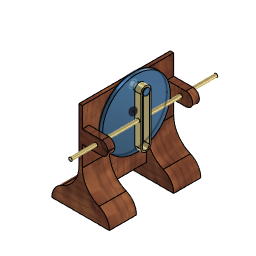
scoci (Autodesk Fusion 360 design; units mm, degrees)
Autodesk Fusion 360 part; units mm, degrees
sketch "Sketch1" plane through (0, 0, 0) normal (1, 0, 0) x (0, 1, 0)
  circle A0 centre (0, 0) radius 50
  circle A1 centre (0, 35) radius 5
  circle A2 centre (0, 0) radius 5
  dimension "d1" = 100
  dimension "d2" = 10
  dimension "d3" = 10
  constraint coincident A0.centre A2.centre
  constraint concentric A0 A2
  measures "d1" diameter of A0
  measures "d2" diameter of A1
  measures "d3" diameter of A2
extrude "Extrude1" add sketch "Sketch1" along normal blind 5 makes body 1
extrude "Extrude2" add sketch "Sketch1" along normal blind 20 contours A1 bodies 1
extrude "Extrude3" add sketch "Sketch1" against normal blind 20 separate body contours A2 makes body 2
extrude "Extrude4" add sketch "Sketch1" along normal blind 5 contours A2 bodies 1 2
ref_plane "WorkPlane1" through (10, 0, 0) normal (1, 0, 0) x (0, 1, 0)
sketch "Sketch2" plane through (10, 0, 0) normal (1, 0, 0) x (0, 1, 0)
  line L0 (-7.4988, -35.1366) -> (-7.5, 34.9999)
  line L1 (7.5, 34.9999) -> (7.5, -35)
  line L2 (-5.25, -35) -> (-5.25, 35)
  line L3 (5.25, -35) -> (5.25, 35)
  arc A0 (-7.4988, -34.8637) -> (7.5, -35) centre (0, -35) ccw
  arc A1 (-5.25, -35) -> (5.25, -35) centre (0, -35) ccw
  arc A2 (7.5, 34.9999) -> (-7.5, 34.9999) centre (0, 35) ccw
  arc A3 (5.25, 35) -> (-5.25, 35) centre (0, 35) ccw
  dimension "d13" = 10.5
  dimension "d14" = 10.5
  dimension "d16" = 15
  constraint concentric A0 A1
  constraint coincident L0.start A0
  constraint tangent L1 A0
  constraint tangent L2 A3
  constraint vertical L2
  constraint tangent L3 A3
  constraint parallel L2 L3
  constraint coincident L0 A0.start
  measures "d13" diameter of A3
  measures "d14" diameter of A1
  measures "d16" diameter of A0
extrude "Extrude5" add sketch "Sketch2" along normal blind 9 separate body makes body 3
sketch "Sketch3" plane through (0, -7.4994, -0.0001) normal (0, -1, -0.000018) x (1, 0, 0)
  line L0 (10, 35) -> (10, -35.1364)
  line L1 (10, -35.1364) -> (19, -35.1364)
  line L2 (19, -35.1364) -> (19, 35)
  line L3 (19, 35) -> (10, 35)
  circle A0 centre (14.92, -0.0682) radius 2.5
  dimension "d19" = 5
  measures "d19" diameter of A0
extrude "Extrude6" add sketch "Sketch3" along normal blind 100 contours A0 bodies 3
sketch "Sketch4" plane through (0, 7.5, 0) normal (0, 1, 0) x (-1, 0, 0)
  line L0 (-10, -35) -> (-10, 34.9999)
  line L1 (-10, 34.9999) -> (-19, 34.9999)
  line L2 (-19, 34.9999) -> (-19, -35)
  line L3 (-19, -35) -> (-10, -35)
  circle A0 centre (-15.0502, -0.0001) radius 2.5
  dimension "d22" = 5
  measures "d22" diameter of A0
extrude "Extrude7" add sketch "Sketch4" along normal blind 100 contours A0 bodies 3
ref_plane "WorkPlane2" through (-5, 0, 0) normal (1, 0, 0) x (0, 1, 0)
sketch "Sketch5" plane through (-5, 0, 0) normal (1, 0, 0) x (0, 1, 0)
  line L0 (65, 40) -> (-70, 40)
  line L1 (-70, 40) -> (-70, -80)
  line L2 (-70, -80) -> (65, -80)
  line L3 (65, -80) -> (65, 40)
  circle A0 centre (0, 0) radius 5.25
  dimension "d26" = 10.5
  constraint horizontal L0
  constraint vertical L1
  constraint horizontal L2
  constraint vertical L3
  constraint coincident A0.centre origin
  measures "d26" diameter of A0
extrude "Extrude8" add sketch "Sketch5" against normal blind 5 separate body makes body 4
sketch "Sketch6" plane through (-5, 0, 0) normal (1, 0, 0) x (0, 1, 0)
  circle A0 centre (0, 0) radius 5.25
  line L0 (65, -80) -> (65, 40)
  line L1 (65, 40) -> (-70, 40)
  line L2 (-70, 40) -> (-70, -80)
  line L3 (-70, -80) -> (65, -80)
  line L4 (-70, -80) -> (-30, -80)
  line L5 (-30, -80) -> (-30, -100)
  line L6 (-30, -100) -> (-70, -100)
  line L7 (-70, -100) -> (-70, -80)
  line L8 (65, -80) -> (25, -80)
  line L9 (25, -80) -> (25, -100)
  line L10 (25, -100) -> (65, -100)
  line L11 (65, -100) -> (65, -80)
  dimension "d29" = 40
  dimension "d30" = 20
  dimension "d31" = 40
  dimension "d32" = 20
  constraint horizontal L4
  constraint vertical L5
  constraint horizontal L6
  constraint vertical L7
  constraint coincident L2.end L3.start
  constraint horizontal L8
  constraint vertical L9
  constraint horizontal L10
  constraint vertical L11
  constraint coincident L0.start L3.end
  measures "d29" distance of L2.end L4.end
  measures "d30" distance of L2.end L6.end
  measures "d31" distance of L0.start L8.end
  measures "d32" distance of L0.start L10.end
extrude "Extrude9" add sketch "Sketch6" against normal blind 45 contours L3 L8 L9 L10 L11 | L3 L4 L5 L6 L7 bodies 4
extrude "Extrude10" add 2 faces at (-50, -56.6667, -86.6667) (-50, 38.3333, -86.6667) along direction (1, 0, 0) blind 85 on bodies 4 bodies 4
fillet "Fillet1" radius 40 4 edges at (-5, -50, -80) (-5, 45, -80) (-10, 45, -80) (-10, -50, -80) on bodies 4
fillet "Fillet2" radius 25 4 edges at (-50, 45, -80) (-50, -50, -80) (35, -50, -80) (35, 45, -80) on bodies 4
sketch "Sketch7" plane through (0, -70, 0) normal (0, -1, 0) x (1, 0, 0)
  arc A0 (35, -100) -> (19.6154, -76.9231) centre (10, -100) ccw
  arc A1 (-5, -40) -> (19.6154, -76.9231) centre (35, -40) ccw
  line L0 (-5, -40) -> (-5, 40)
  line L1 (-5, 40) -> (-10, 40)
  line L2 (-10, 40) -> (-10, -40)
  arc A2 (-34.6154, -76.9231) -> (-10, -40) centre (-50, -40) ccw
  arc A3 (-34.6154, -76.9231) -> (-50, -100) centre (-25, -100) ccw
  line L3 (-50, -100) -> (35, -100)
  line L4 (-5, 9.928) -> (24.1986, 9.928)
  line L5 (33, 0.036) -> (33, -0.036)
  line L6 (23.036, -10) -> (-5, -10)
  line L7 (-5, -10) -> (-5, 9.928)
  circle A4 centre (15, 0) radius 2.75
  arc A5 (22.964, -10) -> (21.8014, 9.928) centre (23, 0) ccw
  dimension "d39" = 5.5
  constraint horizontal L4
  constraint vertical L5
  constraint horizontal L6
  constraint vertical L7
  constraint coincident L0 L4.start
  constraint coincident L4 A5.end
  constraint coincident L6 A5.start
  constraint coincident A5 L4.end
  constraint coincident A5 L5.start
  constraint coincident A5 L5.end
  constraint coincident A5 L6.start
  measures "d39" diameter of A4
extrude "Extrude11" add sketch "Sketch7" against normal blind 10 contours L0 L4 L5 L6 L7 A5 bodies 4
sketch "Sketch8" plane through (0, 65, 0) normal (0, 1, 0) x (-1, 0, 0)
  arc A0 (-19.6154, -76.9231) -> (-35, -100) centre (-10, -100) ccw
  line L0 (-35, -100) -> (50, -100)
  arc A1 (50, -100) -> (34.6154, -76.9231) centre (25, -100) ccw
  arc A2 (10, -40) -> (34.6154, -76.9231) centre (50, -40) ccw
  line L1 (10, -40) -> (10, 40)
  line L2 (10, 40) -> (5, 40)
  line L3 (5, 40) -> (5, -40)
  arc A3 (-19.6154, -76.9231) -> (5, -40) centre (-35, -40) ccw
  line L4 (10, 10) -> (-23.0017, 10)
  line L5 (-23, -10) -> (10, -10)
  line L6 (10, -10) -> (10, 10)
  circle A4 centre (-15, 0) radius 2.75
  arc A5 (-22.9983, 10) -> (-23, -10) centre (-23, 0) ccw
  dimension "d42" = 5.5
  constraint horizontal L4
  constraint horizontal L5
  constraint vertical L6
  constraint coincident L1 L4.start
  constraint coincident L4.end A5
  constraint coincident L4 A5.start
  measures "d42" diameter of A4
extrude "Extrude12" add sketch "Sketch8" against normal blind 10 contours L3 L4 L5 A5 bodies 4
copy_body "Body->Comp1" bodies 4 removing the originals makes body 5 in component "suport"
copy_body "Body->Comp2" bodies 3 removing the originals makes body 6 in component "chestie"
copy_body "Body->Comp3" bodies 1 removing the originals makes body 7 in component "rotita"
component "suport" placed x (1, 0, 0) y (0, 1, 0) z (0, 0, 1) at (0, 0, 0)
component "chestie" placed x (1, 0, 0) y (0, 1, 0) z (0, 0, 1) at (0, 0, 0)
component "rotita" placed x (1, 0, 0) y (0, 1, 0) z (0, 0, 1) at (0, 0, 0)
